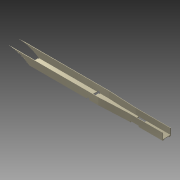
# Autodesk Inventor part: 载板下弹片内3
Saved by Autodesk Inventor 2015 (Build 190159000, 159)
## iProperties
Created: 2017-05-16
Part Number: 载板下弹片内3
Material: 常规
Document SubType Name: Modeling
Designer: Administrator
Density: 1 g/cm^3
Appearance: 镍
Author: Administrator
Autodesk Inventor part; units mm, degrees
ref_plane "YZ Plane" through (0, 0, 0) normal (1, 0, 0) x (0, 1, 0)
ref_plane "XZ Plane" through (0, 0, 0) normal (0, 1, 0) x (-1, 0, 0)
ref_plane "XY Plane" through (0, 0, 0) normal (0, 0, 1) x (1, 0, 0)
sketch "草图1" plane through (0, 0, 0) normal (0, 0, 1) x (1, 0, 0)
  line L0 (-950, 40) -> (0, 40)
  line L1 (0, 40) -> (0, -40)
  line L2 (0, -40) -> (-950, -40)
  line L3 (-950, -40) -> (-950, 40)
  point P0 (0, 0)
  point P1 (0, 0)
  dimension "d0" = 950
  dimension "d1" = 80
  constraints: 8 end point, 2 parallel, 1 coincident, 1 horizontal, 1 midpoint, 1 perpendicular
  measures "d0" distance of L0.start L0.end
  measures "d1" distance of L0.end L1.end
extrude "拉伸1" add sketch "草图1" along normal blind 50
sketch "草图2" plane through (0, -40, 0) normal (1, 0, 0) x (0, 0, -1)
  line L0 (0, 55) -> (-5, 60)
  line L1 (-5, 60) -> (-5, 20)
  line L2 (-5, 20) -> (0, 25)
  line L3 (0, 55) -> (0, 25)
  line L4 (0, 80) -> (0, 0) projected
  line L5 (0, 0) -> (-50, 0) projected
  point P0 (0, 40)
  point P1 (0, 40)
  dimension "d4" = 20
  dimension "d5" = 5
  dimension "d6" = 135
  constraints: 8 end point, 2 midpoint, 1 perpendicular, 1 point on line, 1 vertical
  measures "d4" distance from line of L5 L1.end
  measures "d5" distance between parallel lines of L3 L1
  measures "d6" angle of L4 L0
extrude "拉伸2" cut sketch "草图2" against normal blind 950
sketch "草图4" plane through (0, 0, 50) normal (0, 0, 1) x (1, 0, 0)
  line L0 (0, 30) -> (-250, 30)
  line L1 (-250, 30) -> (-450, 40)
  line L2 (0, 40) -> (-950, 40) projected
  line L3 (-450, 40) -> (0, 40)
  line L4 (0, 40) -> (0, 30)
  line L5 (0, -40) -> (-450, -40)
  line L6 (-950, -40) -> (0, -40) projected
  line L7 (-450, -40) -> (-250, -30)
  line L8 (-250, -30) -> (0, -30)
  line L9 (0, -30) -> (0, -40)
  point P0 (0, 0)
  dimension "d18" = 10
  dimension "d19" = 10
  dimension "d20" = 250
  dimension "d21" = 250
  dimension "d22" = 200
  dimension "d23" = 200
  constraints: 16 end point, 3 point on line, 2 perpendicular, 1 collinear, 1 horizontal, 1 parallel
  measures "d18" distance between parallel lines of L5 L8
  measures "d19" distance between parallel lines of L2 L0
  measures "d20" distance of L0.start L0.end
  measures "d21" distance of L7.end L8.end
  measures "d22" horizontal distance of L0.end L1.end
  measures "d23" horizontal distance of L7.end L5.end
extrude "拉伸4" cut sketch "草图4" against normal blind 50
shell "抽壳2" thickness 3 removed faces 3 at (-783.3333, 13.3333, 50) at (0, 6.6667, 35) at (-950, 6.6667, 35)
sketch "草图5" plane through (-950, 27.2426, 8) normal (0, 0, 1) x (1, 0, 0)
  circle A0 centre (925, -27.2426) radius 2.5
  line L0 (500, 12.7574) -> (0, 12.7574) projected
  point P0 (950, -27.2426)
  dimension "d27" = 5
  dimension "d28" = 25
  dimension "d29" = 40
  constraints: 1 centre point
  measures "d27" diameter of A0
  measures "d28" distance of point (950, -27.243) A0.centre
  measures "d29" distance from line of L0 A0.centre
extrude "拉伸5" cut sketch "草图5" against normal through all
pattern_linear "矩形阵列2" count 10 spacing 100 along (-1, 0, 0) of "拉伸5"
sketch "草图6" plane through (-950, 40, 50) normal (0, 1, 0) x (1, 0, 0)
  arc A0 (414, 47.5) -> (436, 47.5) centre (425, 47.5) ccw
  line L0 (0, 50) -> (500, 50) projected
  line L1 (950, 50) -> (950, 0) projected
  line L2 (414, 47.5) -> (414, 50)
  line L3 (436, 47.5) -> (436, 50)
  line L4 (436, 50) -> (414, 50)
  dimension "d35" = 22
  dimension "d36" = 2.5
  dimension "d37" = 525
  constraints: 6 end point, 2 point on circle, 2 point on line, 2 tangent, 1 centre point, 1 collinear, 1 perpendicular, 1 vertical
  measures "d35" diameter of A0
  measures "d36" distance from line of L0 A0.centre
  measures "d37" distance from line of L1 A0.centre
extrude "拉伸6" cut sketch "草图6" against normal blind 80
sketch "草图7" plane through (-250, 30, 50) normal (0, 1, 0) x (1, 0, 0)
  line L0 (22, 50) -> (78, 50)
  line L1 (78, 50) -> (78, 42)
  line L2 (78, 42) -> (22, 42)
  line L3 (22, 42) -> (22, 50)
  line L4 (250, 50) -> (250, 0) projected
  line L5 (0, 50) -> (250, 50) projected
  dimension "d40" = 56
  dimension "d41" = 172
  dimension "d42" = 8
  dimension "d43" = 8
  constraints: 8 end point, 2 parallel, 1 horizontal, 1 perpendicular
  measures "d40" distance of L1.end L2.end
  measures "d41" distance between parallel lines of L4 L1
  measures "d42" distance between parallel lines of L5 L2
  measures "d43" distance of L0.end L1.end
extrude "拉伸7" cut sketch "草图7" against normal blind 80
sketch "草图8" plane through (-950, 40, 0) normal (-1, 0, 0) x (0, 0, 1)
  line L0 (50, 0) -> (0, 0) projected
  line L1 (50, -3) -> (0, -3)
  line L2 (0, -3) -> (0, 0)
  line L3 (0, 0) -> (50, 0)
  line L4 (50, 0) -> (50, -3)
  line L5 (0, -80) -> (50, -80) projected
  line L6 (50, -80) -> (0, -80)
  line L7 (0, -80) -> (0, -77)
  line L8 (0, -77) -> (50, -77)
  line L9 (50, -77) -> (50, -80)
  line L10 (50, -77) -> (50, -80) projected
  line L11 (50, -77) -> (3, -77) projected
  line L12 (0, -25) -> (0, 0) projected
  point P0 (0, -40)
  constraints: 16 end point, 5 collinear, 4 parallel, 2 horizontal, 2 perpendicular, 1 point on line
extrude "拉伸8" add sketch "草图8" along normal blind 150
sketch "草图10" plane through (-450, 40, 50) normal (0, 1, 0) x (1, 0, 0)
  arc A0 (-650, 0) -> (-500, 50) centre (-650, 250) ccw
  line L0 (0, 0) -> (-650, 0) projected
  line L1 (-650, 0) -> (-650, 50)
  line L2 (-650, 50) -> (-500, 50)
  point P0 (450, 50)
  constraints: 4 end point, 2 point on circle, 1 centre point, 1 perpendicular, 1 tangent, 1 vertical
extrude "拉伸9" cut sketch "草图10" against normal through all
fillet "圆角2" radius 3 2 edges at (-1020.9431, -40, 37.1708) (-1020.9431, 40, 37.1708)
